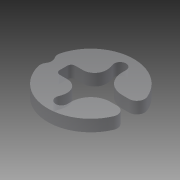
# Autodesk Inventor part: 020914 Aft Middle Endcap
Saved by Autodesk Inventor 2015 (Build 190159000, 159)
## iProperties
Created: 2013-05-23
Part Number: 020914 Aft Middle Endcap
Material: Polycarbonate, Clear
Document SubType Name: Modeling
Designer: Eric
Density: 1.2 g/cm^3
Mass: 0.890235 g
Surface Area: 8.2204 cm^2
Volume: 0.741863 cm^3
Appearance: Polycarbonate - Clear
Author: Eric
Autodesk Inventor part; units mm, degrees
ref_plane "YZ Plane" through (0, 0, 0) normal (1, 0, 0) x (0, 1, 0)
ref_plane "XZ Plane" through (0, 0, 0) normal (0, 1, 0) x (-1, 0, 0)
ref_plane "XY Plane" through (0, 0, 0) normal (0, 0, 1) x (1, 0, 0)
sketch "Sketch1" plane through (0, 0, 0) normal (0, 0, 1) x (1, 0, 0)
  arc A0 (1.5, 7.5) -> (-1.3846, 6.9231) centre (0, 7.5) ccw
  arc A1 (-1.3846, -6.9231) -> (1.5, -7.5) centre (0, -7.5) ccw
  arc A2 (-10.3524, -1.1528) -> (-10.356, 1.1198) centre (-12, -0.0191) ccw
  arc A3 (10.1342, 4.2777) -> (-10.6479, 2.7607) centre (0, 0) ccw
  arc A4 (-10.6391, -2.7946) -> (10.134, -4.278) centre (0, 0) ccw
  arc A5 (-10.6479, 2.7607) -> (-10.356, 1.1198) centre (-8.7119, 2.2588) ccw
  arc A6 (-10.3524, -1.1528) -> (-10.6391, -2.7946) centre (-8.7047, -2.2865) ccw
  arc A7 (-1, 5) -> (-1.3846, 6.9231) centre (-6, 5) ccw
  arc A8 (-1.3846, -6.9231) -> (-1, -5) centre (-6, -5) ccw
  line L0 (1.5, 7.5) -> (1.5, 6.5)
  line L1 (1.4995, -6.5) -> (1.4995, -7.5382)
  line L2 (6.4997, -1.5002) -> (8.2915, -1.5002)
  line L3 (6.4998, 1.5) -> (8.2915, 1.4999)
  arc A9 (6.4997, -1.5002) -> (1.4995, -6.5) centre (6.4995, -6.5002) ccw
  arc A10 (1.5, 6.5) -> (6.4998, 1.5) centre (6.5, 6.5) ccw
  arc A11 (10.134, -4.278) -> (8.2915, -1.5002) centre (8.2915, -3.5002) ccw
  arc A12 (8.2915, 1.4999) -> (10.1342, 4.2777) centre (8.2916, 3.4999) ccw
  line L4 (-6, 2) -> (-4, 2)
  line L5 (-4, -2) -> (-6, -2)
  line L6 (-7, -1) -> (-7, 1)
  arc A13 (-6, 2) -> (-7, 1) centre (-6, 1) ccw
  arc A14 (-7, -1) -> (-6, -2) centre (-6, -1) ccw
  line L7 (-1, -5) -> (-1, -5)
  line L8 (-1, 5) -> (-1, 5)
  arc A15 (-4, 2) -> (-1, 5) centre (-4, 5) ccw
  arc A16 (-1, -5) -> (-4, -2) centre (-4, -5) ccw
  point P0 (10.8972, -1.5003)
  point P1 (10.8973, 1.4999)
  point P2 (1.5, 1.5002)
  point P3 (1.4997, -1.5)
  point P4 (-1, -6.382)
  point P5 (-1, 6.382)
  point P6 (-7, 2)
  point P7 (-7, -2)
  point P8 (-4.7429, 0)
  dimension "d5" = 3
  dimension "d6" = 3
  dimension "d7" = 15
  dimension "d18" = 7.5
  dimension "d20" = 4
  dimension "d21" = 12
  dimension "d22" = 2
  dimension "d26" = 5
  dimension "d27" = 5
  dimension "d28" = 2
  dimension "d30" = 4
  dimension "d31" = 1
  dimension "d32" = 3
  dimension "d33" = 7
  constraints: 39 point on circle, 28 tangent, 18 end point, 17 centre point, 10 point on line, 6 equal radius, 2 parallel, 1 coincident, 1 horizontal, 1 horizontal alignment, 1 perpendicular
  measures "d5" diameter of A0
  measures "d6" diameter of A1
  measures "d7" distance of A1.centre A0.centre
  measures "d18" distance of point (0, 0) A0.centre
  measures "d20" diameter of A2
  measures "d21" distance of point (0, 0) A2.centre
  measures "d22" radius of A5
  measures "d26" radius of A7
  measures "d27" radius of A9
  measures "d28" radius of A11
  measures "d30" distance of point (-7, -2) point (-7, 2)
  measures "d31" radius of A13
  measures "d32" radius of A15
  measures "d33" distance from line of A3.centre L6
extrude "Extrusion2" add sketch "Sketch1" along normal blind 3
body "Solid2"
